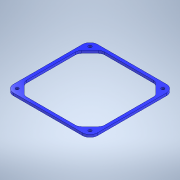
# Autodesk Inventor part: Spacer
Saved by Autodesk Inventor 2020.5 (Build 245400000, 400)
## iProperties
Created: 2024-02-14
Part Number: Spacer
Material: Generic
Document SubType Name: Modeling
Designer: aivel
Density: 1 g/cm^3
Appearance: Blue - Wall Paint - Glossy
Author: aivel
Autodesk Inventor part; units mm, degrees
ref_plane "YZ Plane" through (0, 0, 0) normal (1, 0, 0) x (0, 1, 0)
ref_plane "XZ Plane" through (0, 0, 0) normal (0, 1, 0) x (-1, 0, 0)
ref_plane "XY Plane" through (0, 0, 0) normal (0, 0, 1) x (1, 0, 0)
sketch "Sketch1" plane through (0, 0, 0) normal (0, 1, 0) x (-1, 0, 0)
  line L0 (-10.0391, 0) -> (-100.3906, 0)
  line L1 (-110.4297, -10.0391) -> (-110.4297, -100.3906)
  line L2 (-100.3906, -110.4297) -> (-10.0391, -110.4297)
  line L3 (0, -100.3906) -> (0, -10.0391)
  arc A0 (-10.0391, -110.4297) -> (0, -100.3906) centre (-10.0391, -100.3906) ccw
  arc A1 (-110.4297, -100.3906) -> (-100.3906, -110.4297) centre (-100.3906, -100.3906) ccw
  arc A2 (-100.3906, 0) -> (-110.4297, -10.0391) centre (-100.3906, -10.0391) ccw
  arc A3 (0, -10.0391) -> (-10.0391, 0) centre (-10.0391, -10.0391) ccw
  line L4 (-23.0414, -4.0156) -> (-87.3883, -4.0156)
  line L5 (-106.4141, -23.0414) -> (-106.4141, -87.3883)
  line L6 (-87.3883, -106.4141) -> (-23.0414, -106.4141)
  line L7 (-4.0156, -87.3883) -> (-4.0156, -23.0414)
  circle A4 centre (-7.3285, -7.3285) radius 2.0078
  circle A5 centre (-7.3285, -103.1012) radius 2.0078
  circle A6 centre (-103.1012, -103.1012) radius 2.0078
  circle A7 centre (-103.1012, -7.3285) radius 2.0078
  line L8 (-6.3588, -17.3846) -> (-17.3846, -6.3588)
  line L9 (-93.0451, -6.3588) -> (-104.0709, -17.3846)
  line L10 (-104.0709, -93.0451) -> (-93.0451, -104.0709)
  line L11 (-17.3846, -104.0709) -> (-6.3588, -93.0451)
  arc A8 (-17.3846, -6.3588) -> (-23.0414, -4.0156) centre (-23.0414, -12.0156) ccw
  arc A9 (-4.0156, -23.0414) -> (-6.3588, -17.3846) centre (-12.0156, -23.0414) ccw
  arc A10 (-6.3588, -93.0451) -> (-4.0156, -87.3883) centre (-12.0156, -87.3883) ccw
  arc A11 (-23.0414, -106.4141) -> (-17.3846, -104.0709) centre (-23.0414, -98.4141) ccw
  arc A12 (-93.0451, -104.0709) -> (-87.3883, -106.4141) centre (-87.3883, -98.4141) ccw
  arc A13 (-106.4141, -87.3883) -> (-104.0709, -93.0451) centre (-98.4141, -87.3883) ccw
  arc A14 (-104.0709, -17.3846) -> (-106.4141, -23.0414) centre (-98.4141, -23.0414) ccw
  arc A15 (-87.3883, -4.0156) -> (-93.0451, -6.3588) centre (-87.3883, -12.0156) ccw
  point P0 (0, 0)
  point P1 (-4.0156, -4.0156)
  point P2 (-106.4141, -106.4141)
  point P3 (-106.4141, -4.0156)
  point P4 (-4.0156, -106.4141)
  point P5 (-4.0156, -19.7277)
  point P6 (-19.7277, -4.0156)
  point P7 (-55.2148, -55.2148)
  point P8 (-90.702, -4.0156)
  point P9 (-106.4141, -19.7277)
  point P10 (-106.4141, -90.702)
  point P11 (-90.702, -106.4141)
  point P12 (-19.7277, -106.4141)
  point P13 (-4.0156, -90.702)
  dimension "d25" = 360
  constraints: 24 end point, 24 point on circle, 24 tangent, 20 point on line, 16 centre point, 10 equal radius, 4 parallel, 2 horizontal, 2 perpendicular, 13 other
extrude "Extrusion1" add sketch "Sketch1" along normal blind 3.2
body "Solid1"
